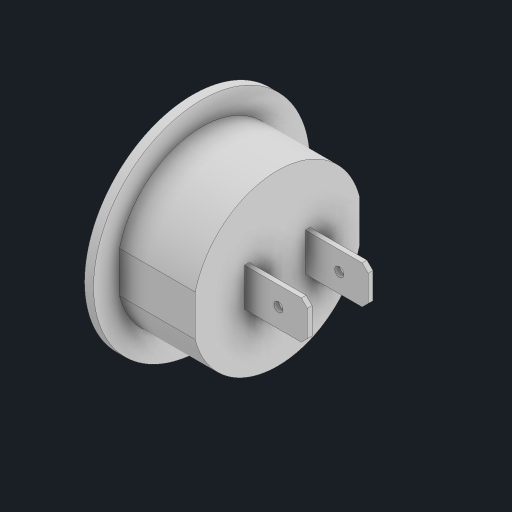
# Autodesk Inventor part: 24vVoltMeter
Saved by Autodesk Inventor 2024 (Build 280153000, 153)
## iProperties
Created: 2023-12-09
Part Number: 24vVoltMeter
Material: Generic
Document SubType Name: Modeling
Designer: 16155
Density: 1 g/cm^3
Appearance: Default
Author: 16155
Autodesk Inventor part; units mm, degrees
ref_plane "YZ Plane" through (0, 0, 0) normal (1, 0, 0) x (0, 1, 0)
ref_plane "XZ Plane" through (0, 0, 0) normal (0, 1, 0) x (-1, 0, 0)
ref_plane "XY Plane" through (0, 0, 0) normal (0, 0, 1) x (1, 0, 0)
sketch "Sketch1" plane through (0, 0, 0) normal (1, 0, 0) x (0, 1, 0)
  circle A0 centre (0, 0) radius 18.125
  dimension "d0" = 36.25
  constraints: 1 centre point, 1 coincident
  measures "d0" diameter of A0
extrude "Extrusion1" add sketch "Sketch1" along normal blind 1.5
sketch "Sketch2" plane through (0, 0, 0) normal (0, 1, 0) x (-1, 0, 0)
  line L0 (0, 0) -> (3.5, 0)
  line L1 (0, 18.125) -> (0, -18.125) projected
  arc A0 (0, -18.125) -> (3.5, 0) centre (-64.8658, 3.8012) ccw
  line L2 (0, 0) -> (0, -18.125)
  line L3 (17.9095, 0) -> (-78.6617, 0) projected
  dimension "d3" = 3.5
  constraints: 4 end point, 2 point on circle, 1 centre point, 1 collinear, 1 horizontal
  measures "d3" distance of L0.start L0.end
revolve "Revolution1" add sketch "Sketch2" angle 360 about axis through (-10, 0, 0) along (1, 0, 0)
sketch "Sketch3" plane through (1.5, 0, 0) normal (1, 0, 0) x (0, 0, -1)
  circle A0 centre (0, 0) radius 14.2
  line L0 (-13.7745, 3.45) -> (13.7745, 3.45)
  line L1 (13.7745, 3.45) -> (13.7745, -3.45)
  line L2 (13.7745, -3.45) -> (-13.7745, -3.45)
  line L3 (-13.7745, -3.45) -> (-13.7745, 3.45)
  line L4 (-13.7745, 3.45) -> (13.7745, -3.45) construction
  line L5 (13.7745, 3.45) -> (-13.7745, -3.45) construction
  dimension "d5" = 28.4
  dimension "d6" = 6.9
  constraints: 12 end point, 2 midpoint, 2 parallel, 1 coincident, 1 horizontal, 1 perpendicular, 3 other
  measures "d6" distance of L0.end L1.end
extrude "Extrusion2" add sketch "Sketch3" along normal blind 12.7 contours L0 A0 | L1 L2 L3 L0 | A0 L2
sketch "Sketch4" plane through (14.2, 0, 0) normal (1, 0, 0) x (0, 0, -1)
  line L0 (-5.5, -3.2) -> (5.5, -3.2)
  line L1 (5.5, -3.2) -> (5.5, 3.2)
  line L2 (5.5, 3.2) -> (-5.5, 3.2)
  line L3 (-5.5, 3.2) -> (-5.5, -3.2)
  line L4 (-5.5, -3.2) -> (5.5, 3.2) construction
  line L5 (5.5, -3.2) -> (-5.5, 3.2) construction
  line L6 (-4.7, -3.2) -> (4.7, -3.2)
  line L7 (4.7, -3.2) -> (4.7, 3.2)
  line L8 (4.7, 3.2) -> (-4.7, 3.2)
  line L9 (-4.7, 3.2) -> (-4.7, -3.2)
  line L10 (-4.7, -3.2) -> (4.7, 3.2) construction
  line L11 (4.7, -3.2) -> (-4.7, 3.2) construction
  point P0 (0, 0)
  dimension "d9" = 11
  dimension "d10" = 6.4
  dimension "d11" = 9.4
  constraints: 24 end point, 4 midpoint, 4 parallel, 2 horizontal, 2 perpendicular, 1 point on line
  measures "d9" distance of L1.end L2.end
  measures "d10" distance of L0.end L1.end
  measures "d11" distance between parallel lines of L9 L7
extrude "Extrusion3" add sketch "Sketch4" along normal blind 10.5 contours L3 L2 L9 L0 | L7 L2 L1 L0
chamfer "Chamfer1" distance 1 angle 45 4 edges at (24.7, 3.2, -5.1) (24.7, -3.2, -5.1) (24.7, -3.2, 5.1) (24.7, 3.2, 5.1)
sketch "Sketch5" plane through (14.2, -3.2, 5.5) normal (0, 0, 1) x (1, 0, 0)
  line L0 (0, 0) -> (0, 6.4) projected
  line L1 (0, 3.2) -> (5.68, 3.2)
  circle A0 centre (5.68, 3.2) radius 0.75
  point P0 (-14.2, 3.2)
  dimension "d17" = 5.68
  dimension "d18" = 1.5
  constraints: 2 end point, 1 centre point, 1 coincident, 1 horizontal, 1 midpoint
  measures "d17" distance of L1.start L1.end
  measures "d18" diameter of A0
extrude "Extrusion4" cut sketch "Sketch5" against normal through all
body "Solid1"
